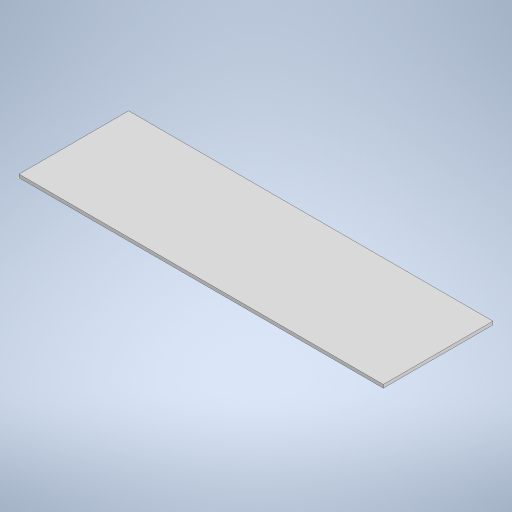
# Autodesk Inventor part: chapinha_garra
Saved by Autodesk Inventor 2024 (Build 280153000, 153)
## iProperties
Created: 2024-10-14
Part Number: chapinha_garra
Material: Genérico
Document SubType Name: Modeling
Designer: robof
Density: 1 g/cm^3
Appearance: Padrão
Author: robof
Autodesk Inventor part; units mm, degrees
ref_plane "YZ Plane" through (0, 0, 0) normal (1, 0, 0) x (0, 1, 0)
ref_plane "XZ Plane" through (0, 0, 0) normal (0, 1, 0) x (-1, 0, 0)
ref_plane "XY Plane" through (0, 0, 0) normal (0, 0, 1) x (1, 0, 0)
sketch "Esboço1" plane through (0, 0, 0) normal (0, 1, 0) x (-1, 0, 0)
  line L0 (0, 0) -> (-113, 0)
  line L1 (-113, 0) -> (-113, -34)
  line L2 (-113, -34) -> (0, -34)
  line L3 (0, -34) -> (0, 0)
  line L4 (0, 0) -> (-7, 0)
  line L5 (0, -11) -> (0, 0)
  circle A0 centre (-7, -11) radius 2.25
  circle A1 centre (-7, -23) radius 2.25
  circle A2 centre (-31, -11) radius 2.25
  circle A3 centre (-31, -23) radius 2.25
  line L6 (-56.5, 0) -> (-56.5, -13.25)
  circle A4 centre (-106, -11) radius 2.25
  circle A5 centre (-106, -23) radius 2.25
  circle A6 centre (-82, -23) radius 2.25
  circle A7 centre (-82, -11) radius 2.25
  circle A8 centre (-7, -11) radius 3.5
  circle A9 centre (-7, -23) radius 3.5
  circle A10 centre (-31, -23) radius 3.5
  circle A11 centre (-31, -11) radius 3.5
  circle A12 centre (-106, -11) radius 3.5
  circle A13 centre (-106, -23) radius 3.5
  circle A14 centre (-82, -23) radius 3.5
  circle A15 centre (-82, -11) radius 3.5
  dimension "d0" = 113
  dimension "d1" = 34
  dimension "d6" = 7
  dimension "d7" = 7
  dimension "d8" = 7
  dimension "d9" = 7
  constraints: 16 centre point, 14 end point, 8 symmetric about line, 5 coincident, 2 horizontal, 2 parallel, 1 midpoint, 1 perpendicular, 1 vertical, 7 other
  measures "d0" distance of L2.end L1.end
  measures "d1" distance of L1.end L0.end
  measures "d6" diameter of A8
  measures "d7" diameter of A9
  measures "d8" diameter of A10
  measures "d9" diameter of A11
extrude "Extrusão1" add sketch "Esboço1" along normal blind 1 contours L3 L2 L1 L0
sketch "Esboço2" plane through (0, 1, 0) normal (0, 1, 0) x (1, 0, 0)
  circle A0 centre (7, 11) radius 3.5 projected
  circle A1 centre (7, 11) radius 3.5
  circle A2 centre (7, 23) radius 3.5 projected
  circle A3 centre (7, 23) radius 3.5
  circle A4 centre (31, 23) radius 3.5 projected
  circle A5 centre (31, 23) radius 3.5
  circle A6 centre (31, 11) radius 3.5 projected
  circle A7 centre (31, 11) radius 3.5
  circle A8 centre (82, 23) radius 3.5 projected
  circle A9 centre (82, 23) radius 3.5
  circle A10 centre (106, 23) radius 3.5 projected
  circle A11 centre (106, 23) radius 3.5
  circle A12 centre (106, 11) radius 3.5 projected
  circle A13 centre (106, 11) radius 3.5
  circle A14 centre (82, 11) radius 3.5 projected
  circle A15 centre (82, 11) radius 3.5
  point P0 (0, 0)
  constraints: 8 centre point, 8 coincident
extrude "Extrusão2" add sketch "Esboço2" against normal blind 2 contours A0 | A2 | A4 | A6 | A8 | A14
sketch "Esboço3" plane through (0, 1, 0) normal (0, 1, 0) x (1, 0, 0)
  circle A0 centre (106, 11) radius 3.5 projected
  circle A1 centre (106, 11) radius 3.5
  circle A2 centre (106, 23) radius 3.5 projected
  circle A3 centre (106, 23) radius 3.5
  point P0 (0, 0)
  constraints: 2 centre point, 2 coincident
extrude "Extrusão3" add sketch "Esboço3" against normal blind 2
sketch "Esboço4" plane through (7, -1, -11) normal (0, -1, 0) x (1, 0, 0)
  circle A0 centre (0, 0) radius 3.5 projected
  circle A1 centre (0, 0) radius 2.25
  line L0 (106, -23) -> (-7, -23) projected
  line L1 (49.5, -23) -> (49.5, -11.349)
  line L2 (0, -23) -> (12, -23)
  line L3 (12, -23) -> (12, -13.2533)
  line L4 (-7, -23) -> (-7, 11) projected
  line L5 (-7, -6) -> (6, -6)
  circle A2 centre (0, -12) radius 2.25
  circle A3 centre (24, 0) radius 2.25
  circle A4 centre (24, -12) radius 2.25
  circle A5 centre (99, 0) radius 2.25
  circle A6 centre (99, -12) radius 2.25
  circle A7 centre (75, 0) radius 2.25
  circle A8 centre (75, -12) radius 2.25
  dimension "d16" = 4.5
  dimension "d17" = 12
  constraints: 8 centre point, 8 end point, 7 symmetric about line, 2 midpoint, 2 point on line, 2 vertical, 1 coincident, 1 horizontal, 7 other
  measures "d16" diameter of A1
  measures "d17" distance of L2.start L2.end
extrude "Extrusão4" add sketch "Esboço4" along normal blind 2.5 contours A1 | A2 | A3 | A4 | A5 | A6 | A7 | A8
sketch "Esboço5" plane through (7, -3.5, -11) normal (0, -1, 0) x (1, 0, 0)
  line L0 (0.0116, -1.5787) -> (-1.3614, -0.7993)
  line L1 (-1.3614, -0.7993) -> (-1.373, 0.7793)
  line L2 (-1.373, 0.7793) -> (-0.0116, 1.5787)
  line L3 (-0.0116, 1.5787) -> (1.3614, 0.7993)
  line L4 (1.3614, 0.7993) -> (1.373, -0.7793)
  line L5 (1.373, -0.7793) -> (0.0116, -1.5787)
  line L6 (-7, -23) -> (-7, 11) projected
  circle A0 centre (0, -12) radius 3.5 projected
  line L7 (106, -23) -> (-7, -23) projected
  line L8 (0.0116, -10.4213) -> (-1.3614, -11.2007)
  line L9 (-1.3614, -11.2007) -> (-1.373, -12.7793)
  line L10 (-1.373, -12.7793) -> (-0.0116, -13.5787)
  line L11 (-0.0116, -13.5787) -> (1.3614, -12.7993)
  line L12 (1.3614, -12.7993) -> (1.373, -11.2207)
  line L13 (1.373, -11.2207) -> (0.0116, -10.4213)
  line L14 (23.9884, -1.5787) -> (25.3614, -0.7993)
  line L15 (25.3614, -0.7993) -> (25.373, 0.7793)
  line L16 (25.373, 0.7793) -> (24.0116, 1.5787)
  line L17 (24.0116, 1.5787) -> (22.6386, 0.7993)
  line L18 (22.6386, 0.7993) -> (22.627, -0.7793)
  line L19 (22.627, -0.7793) -> (23.9884, -1.5787)
  line L20 (23.9884, -10.4213) -> (25.3614, -11.2007)
  line L21 (25.3614, -11.2007) -> (25.373, -12.7793)
  line L22 (25.373, -12.7793) -> (24.0116, -13.5787)
  line L23 (22.6386, -12.7993) -> (22.627, -11.2207)
  line L24 (22.627, -11.2207) -> (23.9884, -10.4213)
  line L25 (24.0116, -13.5787) -> (22.6386, -12.7993)
  line L26 (98.9884, -1.5787) -> (100.3614, -0.7993)
  line L27 (100.3614, -0.7993) -> (100.373, 0.7793)
  line L28 (100.373, 0.7793) -> (99.0116, 1.5787)
  line L29 (99.0116, 1.5787) -> (97.6386, 0.7993)
  line L30 (97.6386, 0.7993) -> (97.627, -0.7793)
  line L31 (97.627, -0.7793) -> (98.9884, -1.5787)
  line L32 (98.9884, -10.4213) -> (100.3614, -11.2007)
  line L33 (100.3614, -11.2007) -> (100.373, -12.7793)
  line L34 (100.373, -12.7793) -> (99.0116, -13.5787)
  line L35 (97.6386, -12.7993) -> (97.627, -11.2207)
  line L36 (97.627, -11.2207) -> (98.9884, -10.4213)
  line L37 (99.0116, -13.5787) -> (97.6386, -12.7993)
  line L38 (75.0116, -10.4213) -> (73.6386, -11.2007)
  line L39 (76.373, -11.2207) -> (75.0116, -10.4213)
  line L40 (73.6386, -11.2007) -> (73.627, -12.7793)
  line L41 (76.3614, -12.7993) -> (76.373, -11.2207)
  line L42 (74.9884, -13.5787) -> (76.3614, -12.7993)
  line L43 (73.627, -12.7793) -> (74.9884, -13.5787)
  line L44 (76.373, -0.7793) -> (75.0116, -1.5787)
  line L45 (73.6386, -0.7993) -> (73.627, 0.7793)
  line L46 (76.3614, 0.7993) -> (76.373, -0.7793)
  line L47 (73.627, 0.7793) -> (74.9884, 1.5787)
  line L48 (74.9884, 1.5787) -> (76.3614, 0.7993)
  line L49 (75.0116, -1.5787) -> (73.6386, -0.7993)
  point P0 (0, 0)
  point P1 (24, 0)
  point P2 (24, -12)
  point P3 (99, 0)
  point P4 (75, 0)
  point P5 (75, -12)
  constraints: 96 end point, 13 other
extrude "Extrusão5" cut sketch "Esboço5" against normal blind 1.5 contours L0 L1 L2 L3 L4 L5 | L13 L12 L11 L10 L9 L8 | L19 L18 L17 L16 L15 L14 | L20 L21 L22 L25 L23 L24 | L31 L30 L29 L28 L27 L26 | L32 L33 L34 L37 L35 L36 | L39 L41 L42 L43 L40 L38 | L44 L49 L45 L47 L48 L46
sketch "Esboço6" plane through (0, 0, 0) normal (0, -1, 0) x (1, 0, 0)
  point P0 (0, 0)
